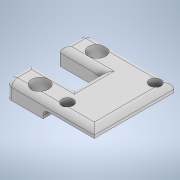
# Autodesk Inventor part: Limit_SwitchMount
Saved by Autodesk Inventor 2021 (Build 250183000, 183)
## iProperties
Created: 2021-03-10
Part Number: Limit_SwitchMount
Material: Generic
Document SubType Name: Modeling
Designer: Jorian Brusind
Density: 1 g/cm^3
Appearance: Default
Author: Jorian Brusind
Autodesk Inventor part; units mm, degrees
ref_plane "YZ Plane" through (0, 0, 0) normal (1, 0, 0) x (0, 1, 0)
ref_plane "XZ Plane" through (0, 0, 0) normal (0, 1, 0) x (-1, 0, 0)
ref_plane "XY Plane" through (0, 0, 0) normal (0, 0, 1) x (1, 0, 0)
sketch "Sketch1" plane through (0, 0, 0) normal (0, 1, 0) x (-1, 0, 0)
  line L0 (0, 0) -> (16, 0)
  line L1 (16, 0) -> (16, -28)
  line L2 (16, -28) -> (0, -28)
  line L3 (0, -28) -> (0, 0)
  dimension "d0" = 16
  dimension "d1" = 28
  constraints: 8 end point, 2 parallel, 1 horizontal, 1 perpendicular
  measures "d0" distance of L1.end L2.end
  measures "d1" distance of L0.end L1.end
extrude "Extrusion1" add sketch "Sketch1" along normal blind 3
sketch "Sketch2" plane through (0, 3, 0) normal (0, 1, 0) x (1, 0, 0)
  circle A0 centre (-3.3, 24.7) radius 2
  circle A1 centre (-12.7, 3.3) radius 2
  line L0 (0, 28) -> (-16, 28) projected
  line L1 (0, 0) -> (0, 28) projected
  line L2 (-16, 28) -> (-16, 0) projected
  line L3 (-16, 0) -> (0, 0) projected
  dimension "d4" = 4
  dimension "d5" = 4
  dimension "d6" = 3.3
  dimension "d7" = 3.3
  dimension "d8" = 3.3
  dimension "d9" = 3.3
  constraints: 2 centre point
  measures "d4" diameter of A0
  measures "d5" diameter of A1
  measures "d6" distance from line of L0 A0.centre
  measures "d7" distance from line of L1 A0.centre
  measures "d8" distance from line of L2 A1.centre
  measures "d9" distance from line of L3 A1.centre
extrude "Extrusion2" cut sketch "Sketch2" against normal blind 3.3 contours A0 | A1
sketch "Sketch10" plane through (0, 3, 0) normal (0, 1, 0) x (1, 0, 0)
  line L0 (-16, 28) -> (-16, 0) projected
  line L1 (-16, 14) -> (-16, 4)
  line L2 (-16, 4) -> (-24, 4)
  line L3 (-16, 0) -> (0, 0) projected
  line L4 (-16, 0) -> (-31, 0)
  line L5 (-31, 0) -> (-31, 9)
  line L6 (-31, 9) -> (-16, 9)
  line L7 (-16, 9) -> (-16, 0)
  line L8 (0, 28) -> (-16, 28) projected
  line L9 (-16, 28) -> (-31, 28)
  line L10 (-31, 28) -> (-31, 19)
  line L11 (-31, 19) -> (-16, 19)
  line L12 (-16, 19) -> (-16, 28)
  dimension "d52" = 10
  dimension "d53" = 8
  dimension "d54" = 15
  dimension "d55" = 9
  dimension "d56" = 15
  dimension "d57" = 9
  constraints: 20 end point, 4 parallel, 3 horizontal, 2 perpendicular, 1 midpoint, 1 point on line
  measures "d52" distance of L1.start L1.end
  measures "d53" distance of L1.end L2.end
  measures "d54" distance of L5.end L6.end
  measures "d55" distance of L4.end L5.end
  measures "d56" distance of L11.end L10.end
  measures "d57" distance of L10.end L9.end
extrude "Extrusion9" add sketch "Sketch10" against normal blind 6
sketch "Sketch11" plane through (0, 3, 0) normal (0, 1, 0) x (1, 0, 0)
  circle A0 centre (-23, 4) radius 3
  circle A1 centre (-23, 24) radius 3
  line L0 (-31, 0) -> (0, 0) projected
  line L1 (-31, 9) -> (-31, 0) projected
  line L2 (-31, 28) -> (-31, 19) projected
  dimension "d60" = 6
  dimension "d61" = 6
  dimension "d62" = 4
  dimension "d63" = 20
  dimension "d64" = 8
  dimension "d65" = 8
  constraints: 2 centre point
  measures "d60" diameter of A0
  measures "d61" diameter of A1
  measures "d62" distance from line of L0 A0.centre
  measures "d63" distance of A1.centre A0.centre
  measures "d64" distance from line of L1 A0.centre
  measures "d65" distance from line of L2 A1.centre
extrude "Extrusion10" cut sketch "Sketch11" against normal through all
sketch "Sketch12" plane through (0, -3, 0) normal (0, -1, 0) x (1, 0, 0)
  line L0 (-16, -9) -> (-31, -9) projected
  line L1 (-16, -9) -> (-18, -9)
  line L2 (-18, -9) -> (-18, 0)
  line L3 (-18, 0) -> (-16, 0)
  line L4 (-16, 0) -> (-16, -9)
  point P0 (0, 0)
  dimension "d68" = 2
  dimension "d69" = 9
  constraints: 8 end point, 2 parallel, 1 horizontal, 1 perpendicular
  measures "d68" distance of L2.end L3.end
  measures "d69" distance of L1.end L2.end
extrude "Extrusion11" cut sketch "Sketch12" against normal blind 3
fillet "Fillet1" radius 2 2 edges at (-16, 0, -23.5) (-18, 0, -4.5)
fillet "Fillet2" radius 2 3 edges at (-15.5, 3, 0) (0, 3, -14) (-15.5, 3, -28)
fillet "Fillet3" radius 2 8 edges at (-31, 2.4142, -27.4142) (-31, -1, -28) (-31, 3, -22.5) (-23.5, 3, -19) (-23.5, 3, -9) (-31, 2.4142, -0.5858) (-31, -1, 0) (-31, 3, -5.5)
fillet "Fillet4" radius 2 2 edges at (-16, 3, -8) (-16, 3, -20)
equation "\"d10\" = d7"
body "Solid1"
